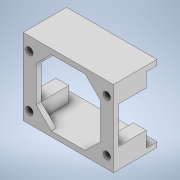
# Autodesk Inventor part: gps_antenna_cover
Saved by Autodesk Inventor 2021 (Build 250183000, 183)
## iProperties
Created: 2020-12-14
Part Number: gps_antenna_cover
Material: Generic
Document SubType Name: Modeling
Designer: Mateusz
Density: 1 g/cm^3
Appearance: Default
Author: Mateusz
Autodesk Inventor part; units mm, degrees
ref_plane "Work Plane1" through (0, 0, 0) normal (0, 0, 1) x (1, 0, 0)
sketch "Sketch1" plane through (0, 0, 0) normal (0, 0, 1) x (1, 0, 0)
  line L0 (0, -26.08) -> (0, 0)
  line L1 (0, 0) -> (-35.6, 0)
  line L2 (-35.6, -26.08) -> (0, -26.08)
  line L3 (-35.6, 0) -> (-35.6, -26.08)
  circle A0 centre (-2.6, -23.48) radius 1.45
  circle A1 centre (-2.6, -3.14) radius 1.45
  circle A2 centre (-33.1, -3.1792) radius 1.45
  circle A3 centre (-33.1, -23.5192) radius 1.45
  line L4 (-30.5, -20.0692) -> (-35.6, -20.0692)
  line L5 (-30.5, -6.6292) -> (-35.6, -6.6292)
  line L6 (-5.1, -5.6288) -> (0, -5.6288)
  line L7 (0, -5.6288) -> (0, 0)
  line L8 (-35.6, -26.08) -> (-35.6, -20.0692)
  line L9 (-35.6, -6.6292) -> (-35.6, 0)
  line L10 (0, -26.08) -> (0, -22.0692)
  line L11 (0, -22.0692) -> (0, -20.0692)
  line L12 (0, -20.0692) -> (-3.1, -20.0692)
  line L13 (-3.1, -20.0692) -> (-5.1, -20.0692)
  line L14 (-17.8, -25.74) -> (-5.1, -25.74)
  line L15 (-5.1, -25.74) -> (-5.1, -0.34)
  line L16 (-5.1, -0.34) -> (-30.5, -0.34)
  line L17 (-30.5, -0.34) -> (-30.5, -25.74)
  line L18 (-30.5, -25.74) -> (-17.8, -25.74)
  line L19 (-5.1, -25.74) -> (-5.1, -26.08)
  line L20 (-5.1, -26.08) -> (0, -26.08)
  line L21 (-30.5, -25.74) -> (-30.5, -26.08)
  line L22 (-35.6, -26.08) -> (-30.5, -26.08)
  line L23 (-30.5, -0.34) -> (-30.5, 0)
  line L24 (-30.5, 0) -> (-35.6, 0)
  line L25 (-5.1, -0.34) -> (-5.1, 0)
  line L26 (-5.1, 0) -> (0, 0)
  line L27 (-5.1, -26.08) -> (-30.5, -26.08)
  line L28 (-30.5, 0) -> (-5.1, 0)
  point P0 (-30.5, 0)
  point P1 (-5.1, 0)
  constraints: 58 end point, 9 point on line, 8 perpendicular, 7 collinear, 4 centre point, 2 parallel, 1 vertical
ref_plane "Work Plane2" through (-34.2906, -29.9214, 10.92) normal (0, 0, 1) x (0.9132, 0.4074, 0)
extrude "Extrusion1" add sketch "Sketch1" along normal up to surface (10.92 mm away) contours L2 L19 L15 L13 L12 L0 | L2 L3 L4 L17 L21 | L6 L15 L25 L1 L0 | L3 L1 L23 L17 L5
sketch "Sketch2" plane through (-5.1, -26.08, 10.92) normal (0, 0, 1) x (1, 0, 0)
  line L0 (-30.5, 0) -> (5.1, 0) projected
  line L1 (5.1, 0) -> (5.1, 26.08) projected
  line L2 (0, 26.08) -> (5.1, 26.08) projected
  line L3 (5.1, 26.08) -> (-30.5, 26.08) projected
  line L4 (-30.5, 26.08) -> (-30.5, 0) projected
  circle A0 centre (-28, 2.5608) radius 1.45 projected
  circle A1 centre (-28, 22.9008) radius 1.45 projected
  circle A2 centre (2.5, 2.6) radius 1.45 projected
  circle A3 centre (2.5, 22.94) radius 1.45 projected
  line L5 (5.1, 0) -> (5.1, -2)
  line L6 (5.1, -2) -> (-30.5, -2)
  line L7 (-30.5, 0) -> (-25.4, 0) projected
  line L8 (-30.5, -2) -> (-30.5, 0)
  line L9 (-30.5, 19.4508) -> (-30.5, 26.08) projected
  line L10 (-30.5, 0) -> (-30.5, 26.08)
  line L11 (-30.5, 26.08) -> (-30.5, 28.08)
  line L12 (-30.5, 28.08) -> (0, 28.08)
  line L13 (0, 28.08) -> (5.1, 28.08)
  line L14 (5.1, 26.08) -> (5.1, 20.4512) projected
  line L15 (5.1, 28.08) -> (5.1, 26.08)
  line L16 (0, 20.4512) -> (0, 26.08) projected
  line L17 (0, 26.08) -> (0, 20.08)
  line L18 (0, 26.08) -> (-6, 26.08)
  line L19 (-6, 26.08) -> (0, 20.08)
  line L20 (-25.4, 19.4508) -> (-25.4, 26.08) projected
  line L21 (-25.4, 26.08) -> (-19.4, 26.08)
  line L22 (-25.4, 26.08) -> (-25.4, 20.08)
  line L23 (-25.4, 20.08) -> (-19.4, 26.08)
  line L24 (-25.4, 0) -> (-19.4, 0)
  line L25 (-25.4, 0) -> (-25.4, 6)
  line L26 (-25.4, 6.0108) -> (-25.4, 0) projected
  line L27 (-25.4, 6) -> (-19.4, 0)
  line L28 (0, 0) -> (-6, 0)
  line L29 (0, 6.0108) -> (0, 0) projected
  line L30 (0, 0) -> (0, 6)
  line L31 (0, 6) -> (-6, 0)
  line L32 (0, 6) -> (0, 20.08)
  line L33 (-25.4, 20.08) -> (-25.4, 6.0108)
  dimension "d19" = 2
  dimension "d20" = 2
  dimension "d21" = 6
  dimension "d22" = 6
  dimension "d23" = 6
  dimension "d24" = 6
  dimension "d25" = 6
  dimension "d26" = 6
  dimension "d27" = 6
  dimension "d28" = 6
  constraints: 44 end point, 10 point on line, 3 collinear, 3 perpendicular, 2 vertical
  measures "d19" distance of L0.end L5.end
  measures "d20" distance of L3.end L11.end
  measures "d21" distance of L2.start L17.end
  measures "d22" distance of L2.start L18.end
  measures "d23" distance of L20.end L21.end
  measures "d24" distance of L20.end L22.end
  measures "d25" distance of L7.end L24.end
  measures "d26" distance of L7.end L25.end
  measures "d27" distance of L28.start L28.end
  measures "d28" distance of L28.start L30.end
extrude "Extrusion2" add sketch "Sketch2" along normal blind 2 contours L4 L3 L20 L33 L26 L25 L0 | L0 L5 L6 L8 | L25 L27 L0 | L11 L12 L13 L15 L2 L3 | L31 L29 L0 | L3 L23 L20 | L0 L29 L32 L17 L16 L2 L1 | L3 L16 L17 L19
ref_plane "Work Plane3" through (-53.6, -42.75, -4.2) normal (0, 0, -1) x (0, 1, 0)
extrude "Extrusion3" add sketch "Sketch2" against normal up to surface (15.12 mm away) contours L0 L5 L6 L8 | L11 L12 L13 L15 L2 L3
body "Solid1"
